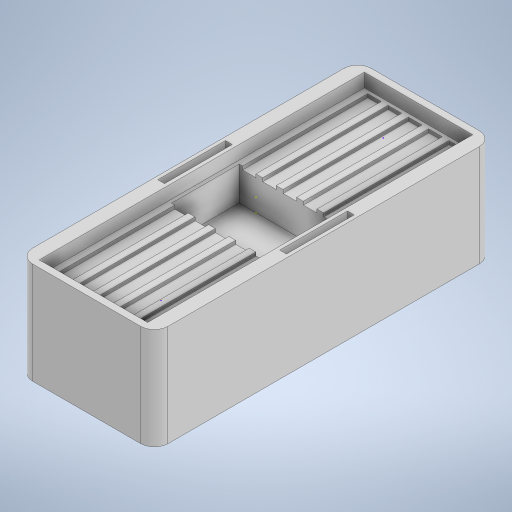
# Autodesk Inventor part: Nadelbox
Saved by Autodesk Inventor 2023.1 (Build 271208000, 208)
## iProperties
Created: 2022-08-08
Part Number: Nadelbox
Material: Generisch
Document SubType Name: Modeling
Designer: schwa
Density: 1 g/cm^3
Appearance: Vorgabe
Author: schwa
Autodesk Inventor part; units mm, degrees
ref_plane "YZ Plane" through (0, 0, 0) normal (1, 0, 0) x (0, 1, 0)
ref_plane "XZ Plane" through (0, 0, 0) normal (0, 1, 0) x (-1, 0, 0)
ref_plane "XY Plane" through (0, 0, 0) normal (0, 0, 1) x (1, 0, 0)
sketch "Skizze1" plane through (0, 0, 0) normal (0, 1, 0) x (-1, 0, 0)
  line L0 (10, 25) -> (-10, 25)
  line L1 (-10, 25) -> (-10, -25)
  line L2 (-10, -25) -> (10, -25)
  line L3 (10, -25) -> (10, 25)
  point P0 (0, 0)
  dimension "d0" = 50
  dimension "d1" = 20
  dimension "d20" = 10
  dimension "d21" = 25
  constraints: 8 end point, 2 parallel, 1 horizontal, 1 perpendicular
  measures "d0" distance of L2.end L0.start
  measures "d1" distance between parallel lines of L1 L3
  measures "d20" distance from line of L3 point (0, 0)
  measures "d21" distance from line of L0 point (0, 0)
extrude "Extrusion1" add sketch "Skizze1" along normal blind 15
sketch "Skizze3" plane through (0, 15, 0) normal (0, 1, 0) x (1, 0, 0)
  line L0 (-8, 24) -> (8, 24)
  line L1 (8, 24) -> (8, -24)
  line L2 (8, -24) -> (-8, -24)
  line L3 (-8, -24) -> (-8, 24)
  line L4 (10, 25) -> (-10, 25) projected
  line L5 (-10, -25) -> (10, -25) projected
  line L6 (10, -25) -> (10, 25) projected
  line L7 (-10, 25) -> (-10, -25) projected
  point P0 (0, 0)
  dimension "d4" = 1
  dimension "d5" = 1
  dimension "d6" = 2
  dimension "d7" = 2
  constraints: 8 end point, 2 parallel, 1 horizontal, 1 perpendicular
  measures "d4" distance between parallel lines of L4 L0
  measures "d5" distance between parallel lines of L2 L5
  measures "d6" distance between parallel lines of L1 L6
  measures "d7" distance between parallel lines of L7 L3
extrude "Extrusion2" cut sketch "Skizze3" against normal blind 2 contours L0 L1 L2 L3
sketch "Skizze4" plane through (0, 13, 0) normal (0, 1, 0) x (1, 0, 0)
  line L0 (-1, 23.5) -> (1, 23.5)
  line L1 (1, 23.5) -> (1, -23.5)
  line L2 (1, -23.5) -> (-1, -23.5)
  line L3 (-1, -23.5) -> (-1, 23.5)
  line L4 (-8, 24) -> (8, 24) projected
  line L5 (8, -24) -> (-8, -24) projected
  line L6 (2, 23.5) -> (4, 23.5)
  line L7 (4, 23.5) -> (4, -23.5)
  line L8 (4, -23.5) -> (2, -23.5)
  line L9 (2, -23.5) -> (2, 23.5)
  line L10 (-7, 23.5) -> (-5, 23.5)
  line L11 (-5, 23.5) -> (-5, -23.5)
  line L12 (-5, -23.5) -> (-7, -23.5)
  line L13 (-7, -23.5) -> (-7, 23.5)
  line L14 (-4, 23.5) -> (-2, 23.5)
  line L15 (-2, 23.5) -> (-2, -23.5)
  line L16 (-2, -23.5) -> (-4, -23.5)
  line L17 (-4, -23.5) -> (-4, 23.5)
  line L18 (5, 23.5) -> (7, 23.5)
  line L19 (7, 23.5) -> (7, -23.5)
  line L20 (7, -23.5) -> (5, -23.5)
  line L21 (5, -23.5) -> (5, 23.5)
  line L22 (-8, -24) -> (-8, 24) projected
  line L23 (8, 24) -> (8, -24) projected
  point P0 (0, 0)
  point P1 (0, -23.5)
  point P2 (0, -24)
  point P3 (6, 23.5)
  dimension "d10" = 2
  dimension "d11" = 0.5
  dimension "d12" = 0.5
  dimension "d33" = 2
  dimension "d34" = 2
  dimension "d35" = 2
  dimension "d36" = 2
  dimension "d37" = 1
  dimension "d38" = 1
  dimension "d39" = 1
  dimension "d40" = 1
  dimension "d41" = 1
  dimension "d42" = 1
  dimension "d50" = 47
  dimension "d51" = 0.5
  dimension "d52" = 0.5
  dimension "d53" = 0.5
  dimension "d54" = 0.5
  dimension "d55" = 47
  constraints: 40 end point, 10 parallel, 5 horizontal, 5 perpendicular, 3 midpoint
  measures "d10" distance of L1.end L2.end
  measures "d11" distance between parallel lines of L4 L0
  measures "d12" distance of point (0, -23.5) point (0, -24)
  measures "d33" distance of L7.end L8.end
  measures "d34" distance of L11.end L13.start
  measures "d35" distance of L15.end L17.start
  measures "d36" distance of L19.end L21.start
  measures "d37" distance between parallel lines of L7 L21
  measures "d38" distance between parallel lines of L1 L9
  measures "d39" distance between parallel lines of L15 L3
  measures "d40" distance between parallel lines of L11 L17
  measures "d41" distance between parallel lines of L22 L13
  measures "d42" distance between parallel lines of L23 L19
  measures "d50" distance between parallel lines of L10 L12
  measures "d51" distance between parallel lines of L5 L12
  measures "d52" distance between parallel lines of L4 L6
  measures "d53" distance between parallel lines of L4 L14
  measures "d54" distance from line of L4 point (6, 23.5)
  measures "d55" distance of L14.start L17.start
sketch "Skizze5" plane through (0, 0, 0) normal (1, 0, 0) x (0, 1, 0)
  point P0 (0, 0)
extrude "Extrusion3" cut sketch "Skizze4" against normal blind 0.5 contours L0 L1 L2 L3 | L6 L7 L8 L9 | L10 L11 L12 L13 | L14 L15 L16 L17 | L18 L19 L20 L21
sketch "Skizze6" plane through (0, 13, 0) normal (0, 1, 0) x (1, 0, 0)
  line L0 (8, 24) -> (8, -24) projected
  point P0 (0, 0)
  point P1 (4.1748, -18.2105)
  point P2 (-0.1937, 19)
  point P3 (8, 0)
  constraints: 1 midpoint
sketch "Skizze8" plane through (0, 15, 0) normal (0, 1, 0) x (1, 0, 0)
  point P0 (0, 0)
sketch "Skizze9" plane through (0, 15, 0) normal (0, 1, 0) x (1, 0, 0)
  line L0 (9.5, 5) -> (8.5, 5)
  line L1 (8.5, 5) -> (8.5, -5)
  line L2 (8.5, -5) -> (9.5, -5)
  line L3 (9.5, -5) -> (9.5, 5)
  line L4 (8, 24) -> (8, -24) construction
  line L5 (-8.5, -5) -> (-9.5, -5)
  line L6 (-9.5, -5) -> (-9.5, 5)
  line L7 (-9.5, 5) -> (-8.5, 5)
  line L8 (-8.5, 5) -> (-8.5, -5)
  line L9 (-10, 25) -> (-10, -25) projected
  point P0 (0, 0)
  point P1 (9, -5)
  point P2 (9.5, 0)
  dimension "d23" = 10
  dimension "d24" = 0.5
  dimension "d25" = 1
  dimension "d26" = 0
  dimension "d29" = 1
  dimension "d30" = 0.5
  constraints: 16 end point, 4 parallel, 2 horizontal, 2 midpoint, 2 perpendicular
  measures "d23" distance from line of point (9, -5) L0
  measures "d24" distance between parallel lines of L4 L1
  measures "d25" distance between parallel lines of L3 L1
  measures "d26" vertical distance of point (0, 0) point (9.5, 0)
  measures "d29" distance of L6.end L7.end
  measures "d30" distance between parallel lines of L9 L6
extrude "Extrusion5" cut sketch "Skizze9" against normal blind 5
sketch "Skizze10" plane through (0, 13, 0) normal (0, 1, 0) x (1, 0, 0)
  line L0 (-7.5, 5) -> (7.5, 5)
  line L1 (7.5, 5) -> (7.5, -5)
  line L2 (7.5, -5) -> (-7.5, -5)
  line L3 (-7.5, -5) -> (-7.5, 5)
  line L4 (-8, -24) -> (-8, 24) projected
  line L5 (8, 24) -> (8, -24) projected
  line L6 (-8, 24) -> (8, 24) projected
  point P0 (0, 0)
  dimension "d43" = 0.5
  dimension "d44" = 0.5
  dimension "d45" = 10
  dimension "d46" = 19
  constraints: 8 end point, 2 parallel, 1 horizontal, 1 perpendicular
  measures "d43" distance between parallel lines of L4 L3
  measures "d44" distance between parallel lines of L1 L5
  measures "d45" distance between parallel lines of L2 L0
  measures "d46" distance between parallel lines of L6 L0
extrude "Extrusion6" cut sketch "Skizze10" against normal blind 5
fillet "Rundung1" radius 2 4 edges at (10, 7.5, 25) (-10, 7.5, 25) (10, 7.5, -25) (-10, 7.5, -25)
